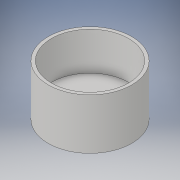
# Autodesk Inventor part: 30-30-FrontSight
Saved by Autodesk Inventor 2019.1 (Build 231200000, 200)
## iProperties
Created: 2018-10-16
Part Number: 30-30-FrontSight
Material: Generic
Document SubType Name: Modeling
Designer: steele
Density: 1 g/cm^3
Appearance: Default
Author: steele
Autodesk Inventor part; units mm, degrees
ref_plane "YZ Plane" through (0, 0, 0) normal (1, 0, 0) x (0, 1, 0)
ref_plane "XZ Plane" through (0, 0, 0) normal (0, 1, 0) x (-1, 0, 0)
ref_plane "XY Plane" through (0, 0, 0) normal (0, 0, 1) x (1, 0, 0)
sketch "Sketch1" plane through (0, 0, 0) normal (0, 1, 0) x (-1, 0, 0)
  circle A0 centre (0, 0) radius 20.955
  dimension "d0" = 41.91
  constraints: 1 centre point, 1 coincident
  measures "d0" diameter of A0
extrude "Extrusion1" add sketch "Sketch1" against normal blind 6.35
sketch "Sketch2" plane through (0, 0, 0) normal (0, 1, 0) x (1, 0, 0)
  circle A0 centre (0, 0) radius 20.955
  circle A1 centre (0, 0) radius 19.3675
  dimension "d3" = 38.735
  dimension "d4" = 41.91
  constraints: 2 centre point, 2 coincident
  measures "d3" diameter of A1
  measures "d4" diameter of A0
extrude "Extrusion2" add sketch "Sketch2" along normal blind 19.05
sketch "Sketch3" plane through (0, -6.35, 0) normal (0, -1, 0) x (1, 0, 0)
  circle A0 centre (0, 0) radius 20.955 construction
  line L0 (20.955, 0) -> (-20.955, 0) construction
  line L1 (16.9505, 3.175) -> (20.3673, 3.175)
  line L2 (20.3673, 3.175) -> (20.3673, 2.0686)
  line L3 (20.3673, 2.0686) -> (19.4565, 2.0686)
  line L4 (19.4565, 2.0686) -> (19.4565, -2.0686)
  line L5 (19.4565, -2.0686) -> (20.3673, -2.0686)
  line L6 (20.3673, -2.0686) -> (20.3673, -3.175)
  line L7 (20.3673, -3.175) -> (16.9505, -3.175)
  line L8 (16.9505, -3.175) -> (16.9505, -2.0686)
  line L9 (16.9505, -2.0686) -> (17.8613, -2.0686)
  line L10 (17.8613, -2.0686) -> (17.8613, 2.0686)
  line L11 (17.8613, 2.0686) -> (16.9505, 2.0686)
  line L12 (16.9505, 2.0686) -> (16.9505, 3.175)
  spline S0 degree 2 poles (10.2248, 0.0051) (10.2248, 0.8954) (11.0019, 2.2951) (11.5936, 2.6707) knots 0 0 0 1 2 2 2
  spline S1 degree 2 poles (11.5936, 2.6707) (12.0876, 2.9897) (13.2506, 3.175) (13.9041, 3.175) knots 0 0 0 1 2 2 2
  line L13 (13.9041, 3.175) -> (15.8904, 3.175)
  line L14 (15.8904, 3.175) -> (15.8904, -3.175)
  line L15 (15.8904, -3.175) -> (13.9247, -3.175)
  spline S2 degree 2 poles (13.9247, -3.175) (13.2558, -3.175) (12.0876, -3.0052) (11.5731, -2.6759) knots 0 0 0 1 2 2 2
  spline S3 degree 2 poles (11.5731, -2.6759) (10.9504, -2.2745) (10.2248, -0.916) (10.2248, 0.0051) knots 0 0 0 1 2 2 2
  spline S4 degree 2 poles (11.8612, -0.0051) (11.8612, -0.6329) (12.2935, -1.5283) (12.736, -1.7805) knots 0 0 0 1 2 2 2
  spline S5 degree 2 poles (12.736, -1.7805) (13.0602, -1.9554) (13.7703, -1.9915) (14.2643, -1.9915) knots 0 0 0 1 2 2 2
  line L16 (14.2643, -1.9915) -> (14.2952, -1.9915)
  line L17 (14.2952, -1.9915) -> (14.2952, 1.9863)
  line L18 (14.2952, 1.9863) -> (14.2643, 1.9863)
  spline S6 degree 2 poles (14.2643, 1.9863) (13.7292, 1.9863) (12.9933, 1.9503) (12.6588, 1.7393) knots 0 0 0 1 2 2 2
  spline S7 degree 2 poles (12.6588, 1.7393) (12.2677, 1.4923) (11.8612, 0.6226) (11.8612, -0.0051) knots 0 0 0 1 2 2 2
  line L19 (7.5953, 3.175) -> (9.103, 3.175)
  line L20 (9.103, 3.175) -> (9.103, 1.4974)
  line L21 (9.103, 1.4974) -> (7.5953, 1.4974)
  line L22 (7.5953, 1.4974) -> (7.5953, 3.175)
  line L23 (7.5953, 0.0618) -> (9.103, 0.0618)
  line L24 (9.103, 0.0618) -> (9.103, -1.6158)
  line L25 (9.103, -1.6158) -> (7.5953, -1.6158)
  line L26 (7.5953, -1.6158) -> (7.5953, 0.0618)
  line L27 (-0.8182, 3.175) -> (3.3757, 3.175)
  line L28 (3.3757, 3.175) -> (3.3757, 2.0686)
  line L29 (3.3757, 2.0686) -> (2.0378, 2.0686)
  line L30 (2.0378, 2.0686) -> (2.0378, -1.2916)
  line L31 (2.0378, -1.2916) -> (3.3757, -1.2916)
  line L32 (3.3757, -1.2916) -> (3.3757, -2.3259)
  spline S8 degree 2 poles (3.3757, -2.3259) (3.0824, -2.3259) (2.5009, -2.4031) (2.3259, -2.4855) knots 0 0 0 1 2 2 2
  spline S9 degree 2 poles (2.3259, -2.4855) (2.1252, -2.5884) (1.8988, -2.9331) (1.8782, -3.1904) knots 0 0 0 1 2 2 2
  line L33 (1.8782, -3.1904) -> (0.4889, -3.1904)
  line L34 (0.4889, -3.1904) -> (0.4889, 2.0686)
  line L35 (0.4889, 2.0686) -> (-0.8182, 2.0686)
  line L36 (-0.8182, 2.0686) -> (-0.8182, 3.175)
  line L37 (-3.4683, 3.175) -> (-1.9606, 3.175)
  line L38 (-1.9606, 3.175) -> (-1.9606, 1.4974)
  line L39 (-1.9606, 1.4974) -> (-3.4683, 1.4974)
  line L40 (-3.4683, 1.4974) -> (-3.4683, 3.175)
  spline S10 degree 2 poles (-9.2471, 1.024) (-9.2471, 1.5232) (-8.9075, 2.3671) (-8.573, 2.6707) knots 0 0 0 1 2 2 2
  spline S11 degree 2 poles (-8.573, 2.6707) (-8.2385, 2.9743) (-7.3226, 3.3088) (-6.6536, 3.3088) knots 0 0 0 1 2 2 2
  spline S12 degree 2 poles (-6.6536, 3.3088) (-5.9435, 3.3036) (-4.9246, 3.0721) (-4.5901, 2.9229) knots 0 0 0 1 2 2 2
  line L41 (-4.5901, 2.9229) -> (-4.5901, 1.5386)
  line L42 (-4.5901, 1.5386) -> (-4.7342, 1.5386)
  spline S13 degree 2 poles (-4.7342, 1.5386) (-4.8577, 1.6055) (-5.1562, 1.7805) (-5.398, 1.8731) knots 0 0 0 1 2 2 2
  spline S14 degree 2 poles (-5.398, 1.8731) (-5.6244, 1.9606) (-6.0927, 2.0789) (-6.3757, 2.0789) knots 0 0 0 1 2 2 2
  spline S15 degree 2 poles (-6.3757, 2.0789) (-6.6227, 2.0789) (-7.1991, 1.9554) (-7.374, 1.7908) knots 0 0 0 1 2 2 2
  spline S16 degree 2 poles (-7.374, 1.7908) (-7.5027, 1.6621) (-7.6468, 1.3482) (-7.6468, 1.0858) knots 0 0 0 1 2 2 2
  spline S17 degree 2 poles (-7.6468, 1.0858) (-7.6468, 0.8594) (-7.4615, 0.5403) (-7.3123, 0.4425) knots 0 0 0 1 2 2 2
  spline S18 degree 2 poles (-7.3123, 0.4425) (-7.0962, 0.2985) (-6.4786, 0.2161) (-6.2574, 0.2161) knots 0 0 0 1 2 2 2
  spline S19 degree 2 poles (-6.2574, 0.2161) (-5.9075, 0.2161) (-5.2436, 0.3293) (-5.0018, 0.3911) knots 0 0 0 1 2 2 2
  line L43 (-5.0018, 0.3911) -> (-4.8628, 0.3911)
  line L44 (-4.8628, 0.3911) -> (-4.8628, -3.175)
  line L45 (-4.8628, -3.175) -> (-9.0722, -3.175)
  line L46 (-9.0722, -3.175) -> (-9.0722, -1.976)
  line L47 (-9.0722, -1.976) -> (-6.3706, -1.976)
  line L48 (-6.3706, -1.976) -> (-6.3706, -0.9211)
  spline S20 degree 2 poles (-6.3706, -0.9211) (-6.4992, -0.9314) (-6.8543, -0.9417) (-6.9521, -0.9417) knots 0 0 0 1 2 2 2
  spline S21 degree 2 poles (-6.9521, -0.9417) (-7.41, -0.9417) (-8.1819, -0.7564) (-8.4855, -0.566) knots 0 0 0 1 2 2 2
  spline S22 degree 2 poles (-8.4855, -0.566) (-8.8457, -0.3293) (-9.2471, 0.458) (-9.2471, 1.024) knots 0 0 0 1 2 2 2
  line L49 (-14.9539, 3.175) -> (-10.2866, 3.175)
  line L50 (-10.2866, 3.175) -> (-10.2866, 2.1407)
  spline S23 degree 2 poles (-10.2866, 2.1407) (-10.8784, 1.6673) (-11.8252, 0.8336) (-12.1803, 0.458) knots 0 0 0 1 2 2 2
  spline S24 degree 2 poles (-12.1803, 0.458) (-12.6485, -0.0309) (-13.0654, -0.777) (-13.0654, -1.1681) knots 0 0 0 1 2 2 2
  spline S25 degree 2 poles (-13.0654, -1.1681) (-13.0654, -1.6107) (-12.5353, -2.0841) (-12.0619, -2.0841) knots 0 0 0 1 2 2 2
  spline S26 degree 2 poles (-12.0619, -2.0841) (-11.8201, -2.0841) (-11.3878, -1.9657) (-11.1665, -1.8731) knots 0 0 0 1 2 2 2
  spline S27 degree 2 poles (-11.1665, -1.8731) (-10.9504, -1.7753) (-10.6417, -1.5695) (-10.5645, -1.518) knots 0 0 0 1 2 2 2
  line L51 (-10.5645, -1.518) -> (-10.441, -1.518)
  line L52 (-10.441, -1.518) -> (-10.441, -2.9023)
  spline S28 degree 2 poles (-10.441, -2.9023) (-10.7085, -3.0309) (-11.8509, -3.2985) (-12.381, -3.2985) knots 0 0 0 1 2 2 2
  spline S29 degree 2 poles (-12.381, -3.2985) (-13.513, -3.2985) (-14.676, -2.2899) (-14.676, -1.3791) knots 0 0 0 1 2 2 2
  spline S30 degree 2 poles (-14.676, -1.3791) (-14.676, -0.8182) (-14.146, 0.2624) (-13.5336, 0.8799) knots 0 0 0 1 2 2 2
  spline S31 degree 2 poles (-13.5336, 0.8799) (-13.1477, 1.2607) (-12.4221, 1.8525) (-12.2626, 1.976) knots 0 0 0 1 2 2 2
  line L53 (-12.2626, 1.976) -> (-14.9539, 1.976)
  line L54 (-14.9539, 1.976) -> (-14.9539, 3.175)
  spline S32 degree 2 poles (-20.3725, 1.024) (-20.3725, 1.5232) (-20.0329, 2.3671) (-19.6984, 2.6707) knots 0 0 0 1 2 2 2
  spline S33 degree 2 poles (-19.6984, 2.6707) (-19.3639, 2.9743) (-18.4479, 3.3088) (-17.779, 3.3088) knots 0 0 0 1 2 2 2
  spline S34 degree 2 poles (-17.779, 3.3088) (-17.0688, 3.3036) (-16.05, 3.0721) (-15.7155, 2.9229) knots 0 0 0 1 2 2 2
  line L55 (-15.7155, 2.9229) -> (-15.7155, 1.5386)
  line L56 (-15.7155, 1.5386) -> (-15.8596, 1.5386)
  spline S35 degree 2 poles (-15.8596, 1.5386) (-15.9831, 1.6055) (-16.2815, 1.7805) (-16.5234, 1.8731) knots 0 0 0 1 2 2 2
  spline S36 degree 2 poles (-16.5234, 1.8731) (-16.7498, 1.9606) (-17.2181, 2.0789) (-17.5011, 2.0789) knots 0 0 0 1 2 2 2
  spline S37 degree 2 poles (-17.5011, 2.0789) (-17.7481, 2.0789) (-18.3244, 1.9554) (-18.4994, 1.7908) knots 0 0 0 1 2 2 2
  spline S38 degree 2 poles (-18.4994, 1.7908) (-18.628, 1.6621) (-18.7721, 1.3482) (-18.7721, 1.0858) knots 0 0 0 1 2 2 2
  spline S39 degree 2 poles (-18.7721, 1.0858) (-18.7721, 0.8594) (-18.5869, 0.5403) (-18.4376, 0.4425) knots 0 0 0 1 2 2 2
  spline S40 degree 2 poles (-18.4376, 0.4425) (-18.2215, 0.2985) (-17.604, 0.2161) (-17.3827, 0.2161) knots 0 0 0 1 2 2 2
  spline S41 degree 2 poles (-17.3827, 0.2161) (-17.0328, 0.2161) (-16.369, 0.3293) (-16.1271, 0.3911) knots 0 0 0 1 2 2 2
  line L57 (-16.1271, 0.3911) -> (-15.9882, 0.3911)
  line L58 (-15.9882, 0.3911) -> (-15.9882, -3.175)
  line L59 (-15.9882, -3.175) -> (-20.1975, -3.175)
  line L60 (-20.1975, -3.175) -> (-20.1975, -1.976)
  line L61 (-20.1975, -1.976) -> (-17.4959, -1.976)
  line L62 (-17.4959, -1.976) -> (-17.4959, -0.9211)
  spline S42 degree 2 poles (-17.4959, -0.9211) (-17.6246, -0.9314) (-17.9797, -0.9417) (-18.0774, -0.9417) knots 0 0 0 1 2 2 2
  spline S43 degree 2 poles (-18.0774, -0.9417) (-18.5354, -0.9417) (-19.3073, -0.7564) (-19.6109, -0.566) knots 0 0 0 1 2 2 2
  spline S44 degree 2 poles (-19.6109, -0.566) (-19.9711, -0.3293) (-20.3725, 0.458) (-20.3725, 1.024) knots 0 0 0 1 2 2 2
  constraints: 2 end point, 2 horizontal, 2 point on circle
extrude "Extrusion3" cut sketch "Sketch3" against normal blind 3.175
equation "\"d0\" = outerDiam"
equation "\"d1\" = endCapThickness"
equation "\"d3\" = internalDiam"
equation "\"d4\" = outerDiam"
equation "\"d5\" = length"
equation "\"length\" = 19.05"
equation "\"internalDiam\" = 38.735"
equation "\"wallThickness\" = 1.5875"
equation "\"endCapThickness\" = 6.35"
equation "\"outerDiam\" = internalDiam + 2 * wallThickness"
body "Solid1"
